Autodesk Fusion 360 part; units mm, degrees
(part 2 of 2)
sketch "Sketch38" plane through (0, 15.0006, 0) normal (0, -1, 0) x (1, 0, 0)
  line L0 (-1.1388, 9) -> (-3.0388, 9)
  line L1 (-3.0388, 9) -> (-3.0388, 0.2)
  line L2 (-3.0388, 0.2) -> (-3.0388, -5)
  line L3 (-3.0388, -5) -> (-1.1388, -5)
  line L4 (-1.1388, -5) -> (-1.1388, 9)
  line L5 (-3.7888, -3) -> (-3.0388, -3)
  line L6 (-3.0388, -3) -> (-3.0388, -5)
  line L7 (-3.0388, -5) -> (-3.7888, -3)
  line L8 (61.4612, 9) -> (59.5612, 9)
  line L9 (59.5612, 9) -> (59.5612, -5)
  line L10 (59.5612, -5) -> (61.4612, -5)
  line L11 (61.4612, -5) -> (61.4612, -1.4)
  line L12 (61.4612, -1.4) -> (61.4612, 9)
  line L13 (62.2112, -3) -> (61.4612, -3)
  line L14 (61.4612, -3) -> (61.4612, -5)
  line L15 (61.4612, -5) -> (62.2112, -3)
  dimension "d420" = 2
  dimension "d422" = 2
  constraint horizontal L5
  constraint vertical L6
  constraint coincident L2.end L3.start
  constraint horizontal L13
  constraint vertical L14
  constraint coincident L10.end L11.start
  measures "d420" distance of L2.end L5.end
  measures "d422" distance of L10.end L13.end
extrude "Extrude62" add sketch "Sketch38" against normal up to surface (8 mm away) contours L2 L5 L6 L7 | L11 L13 L14 L15 bodies 2
sketch "Sketch39" plane through (4.9612, 0, 0) normal (-1, 0, 0) x (0, -1, 0)
  line L0 (-52.9006, 9) -> (-54.8006, 9)
  line L1 (-54.8006, 9) -> (-54.8006, 0.2)
  line L2 (-54.8006, 0.2) -> (-54.8006, -5)
  line L3 (-54.8006, -5) -> (-52.9006, -5)
  line L4 (-52.9006, -5) -> (-52.9006, 9)
  line L5 (-55.5506, -3) -> (-54.8006, -3)
  line L6 (-54.8006, -3) -> (-54.8006, -5)
  line L7 (-54.8006, -5) -> (-55.5506, -3)
  dimension "d426" = 2
  constraint horizontal L5
  constraint vertical L6
  constraint coincident L2.end L3.start
  measures "d426" distance of L2.end L5.end
extrude "Extrude63" add sketch "Sketch39" against normal up to surface (8 mm away) contours L2 L5 L6 L7 bodies 2
sketch "Sketch40" plane through (53.4612, 0, 0) normal (1, 0, 0) x (0, 1, 0)
  line L0 (54.8006, 9) -> (52.9006, 9)
  line L1 (52.9006, 9) -> (52.9006, -5)
  line L2 (52.9006, -5) -> (54.8006, -5)
  line L3 (54.8006, -5) -> (54.8006, 0.2)
  line L4 (54.8006, 0.2) -> (54.8006, 9)
  line L5 (55.5506, -3) -> (54.8006, -3)
  line L6 (54.8006, -3) -> (54.8006, -5)
  line L7 (54.8006, -5) -> (55.5506, -3)
  dimension "d430" = 2
  constraint horizontal L5
  constraint vertical L6
  constraint coincident L2.end L3.start
  measures "d430" distance of L2.end L5.end
extrude "Extrude64" add sketch "Sketch40" against normal up to surface (8 mm away) contours L3 L5 L6 L7 bodies 2
sketch "Sketch41" plane through (0, 54.8006, 0) normal (0, -1, 0) x (1, 0, 0)
  line L0 (-2.0388, -7) -> (60.4612, -7)
  line L1 (60.4612, -7) -> (60.4612, -1.6)
  line L2 (60.4612, -1.6) -> (-2.0388, -1.6)
  line L3 (-2.0388, -1.6) -> (-2.0388, -7)
  line L4 (53.4612, -5) -> (53.4612, -3)
  line L5 (53.4612, -3) -> (45.4612, -3)
  line L6 (45.4612, -5) -> (45.4612, -3)
  line L7 (45.4612, -5) -> (53.4612, -5)
  line L8 (12.9612, -3) -> (12.9612, -5)
  line L9 (4.9612, -5) -> (12.9612, -5)
  line L10 (4.9612, -3) -> (12.9612, -3)
  line L11 (4.9612, -5) -> (4.9612, -3)
  line L12 (13.4612, -2.75) -> (4.4612, -2.75)
  line L13 (4.4612, -2.75) -> (4.4612, -5.5)
  line L14 (4.4612, -5.5) -> (13.4612, -5.5)
  line L15 (13.4612, -5.5) -> (13.4612, -2.75)
  line L16 (53.9612, -2.75) -> (44.9612, -2.75)
  line L17 (44.9612, -2.75) -> (44.9612, -5.5)
  line L18 (44.9612, -5.5) -> (53.9612, -5.5)
  line L19 (53.9612, -5.5) -> (53.9612, -2.75)
  dimension "d434" = 0.25
  dimension "d435" = 0.5
  dimension "d436" = 0.5
  dimension "d437" = 0.5
  dimension "d438" = 0.25
  dimension "d439" = 0.5
  dimension "d440" = 0.5
  dimension "d441" = 0.5
  constraint horizontal L12
  constraint vertical L13
  constraint horizontal L14
  constraint vertical L15
  constraint horizontal L16
  constraint vertical L17
  constraint horizontal L18
  constraint vertical L19
  measures "d434" distance of L10 L12
  measures "d435" distance of L9 L14
  measures "d436" distance of L8 L15
  measures "d437" distance of L11 L13
  measures "d438" distance of L5 L16
  measures "d439" distance of L6 L17
  measures "d440" distance of L7 L18
  measures "d441" distance of L4 L19
extrude "Extrude65" cut sketch "Sketch41" against normal blind 1 contours L4 L5 L6 L7 | L8 L9 L10 L11 | L12 L13 L14 L15 | L16 L17 L18 L19 bodies 1
sketch "Sketch42" plane through (61.4612, 0, 0) normal (-1, 0, 0) x (0, -1, 0)
  line L0 (-48.8006, -7) -> (-11.7006, -7)
  line L1 (-11.7006, -7) -> (-11.7006, -1.6)
  line L2 (-11.7006, -1.6) -> (-48.8006, -1.6)
  line L3 (-48.8006, -1.6) -> (-48.8006, -7)
  line L4 (-15.0006, -5) -> (-15.0006, -3)
  line L5 (-15.0006, -3) -> (-23.0006, -3)
  line L6 (-23.0006, -5) -> (-23.0006, -3)
  line L7 (-23.0006, -5) -> (-15.0006, -5)
  line L8 (-14.5006, -2.75) -> (-23.5006, -2.75)
  line L9 (-23.5006, -2.75) -> (-23.5006, -5.5)
  line L10 (-23.5006, -5.5) -> (-14.5006, -5.5)
  line L11 (-14.5006, -5.5) -> (-14.5006, -2.75)
  dimension "d444" = 0.25
  dimension "d445" = 0.5
  dimension "d446" = 0.5
  dimension "d447" = 0.5
  constraint horizontal L8
  constraint vertical L9
  constraint horizontal L10
  constraint vertical L11
  measures "d444" distance of L5 L8
  measures "d445" distance of L7 L10
  measures "d446" distance of L6 L9
  measures "d447" distance of L4 L11
extrude "Extrude66" cut sketch "Sketch42" against normal blind 1 contours L4 L5 L6 L7 | L8 L9 L10 L11 bodies 1
sketch "Sketch43" plane through (-3.0388, 0, 0) normal (1, 0, 0) x (0, 1, 0)
  line L0 (11.7006, -7) -> (48.8006, -7)
  line L1 (48.8006, -7) -> (48.8006, -1.6)
  line L2 (48.8006, -1.6) -> (11.7006, -1.6)
  line L3 (11.7006, -1.6) -> (11.7006, -7)
  line L4 (23.0006, -3) -> (23.0006, -5)
  line L5 (15.0006, -3) -> (23.0006, -3)
  line L6 (15.0006, -5) -> (15.0006, -3)
  line L7 (15.0006, -5) -> (23.0006, -5)
  line L8 (23.5006, -2.75) -> (14.5006, -2.75)
  line L9 (14.5006, -2.75) -> (14.5006, -5.5)
  line L10 (14.5006, -5.5) -> (23.5006, -5.5)
  line L11 (23.5006, -5.5) -> (23.5006, -2.75)
  dimension "d450" = 0.5
  dimension "d451" = 0.5
  dimension "d452" = 0.5
  dimension "d453" = 0.25
  constraint horizontal L8
  constraint vertical L9
  constraint horizontal L10
  constraint vertical L11
  measures "d450" distance of L6 L9
  measures "d451" distance of L7 L10
  measures "d452" distance of L4 L11
  measures "d453" distance of L5 L8
extrude "Extrude67" cut sketch "Sketch43" against normal blind 1 contours L4 L5 L6 L7 | L8 L9 L10 L11 bodies 1
copy_body "Body->Comp6" bodies 1 removing the originals makes body 3 in component "bottom shell"
copy_body "Body->Comp7" bodies 2 removing the originals makes body 4 in component "top shell"
sketch "Sketch44" plane through (63.4612, 0, 0) normal (1, 0, 0) x (0, 1, 0)
  line L0 (0.0006, -9) -> (53.8006, -9)
  line L1 (53.8006, -9) -> (53.8006, 0)
  line L2 (53.8006, 0) -> (0.0006, 0)
  line L3 (0.0006, 0) -> (0.0006, -9)
  line L4 (23.5006, -5.5) -> (23.5006, -2.75)
  line L5 (14.5006, -2.75) -> (14.5006, -5.5)
  line L6 (23.5006, -4.125) -> (14.5006, -4.125)
  point P0 (19.0006, -4.125)
  constraint midpoint L4 L6.start
  constraint midpoint L5 L6.end
  constraint midpoint L6 P0
hole "Hole1" at (63.4612, 19.0006, -4.125) direction (-1, 0, 0) diameter 2 depth 2 tip angle 180 bodies 3 in component "bottom shell"
sketch "Sketch45" plane through (-5.0388, 0, 0) normal (-1, 0, 0) x (0, -1, 0)
  line L0 (-53.8006, -9) -> (-0.0006, -9)
  line L1 (-0.0006, -9) -> (-0.0006, 0)
  line L2 (-0.0006, 0) -> (-53.8006, 0)
  line L3 (-53.8006, 0) -> (-53.8006, -9)
  line L4 (-14.5006, -5.5) -> (-14.5006, -2.75)
  line L5 (-23.5006, -2.75) -> (-23.5006, -5.5)
  line L6 (-23.5006, -4.125) -> (-14.5006, -4.125)
  point P0 (-19.0006, -4.125)
  constraint midpoint L5 L6.start
  constraint midpoint L4 L6.end
  constraint midpoint L6 P0
hole "Hole2" at (-5.0388, 19.0006, -4.125) direction (1, 0, 0) diameter 2 depth 2 tip angle 180 bodies 3 in component "bottom shell"
sketch "Sketch46" plane through (0, 56.8006, 0) normal (0, 1, 0) x (-1, 0, 0)
  line L0 (-60.4612, -9) -> (2.0388, -9)
  line L1 (2.0388, -9) -> (2.0388, 0)
  line L2 (2.0388, 0) -> (-60.4612, 0)
  line L3 (-60.4612, 0) -> (-60.4612, -9)
  line L4 (-13.4612, -2.75) -> (-13.4612, -5.5)
  line L5 (-4.4612, -5.5) -> (-4.4612, -2.75)
  line L6 (-53.9612, -2.75) -> (-53.9612, -5.5)
  line L7 (-44.9612, -5.5) -> (-44.9612, -2.75)
  line L8 (-53.9612, -4.125) -> (-44.9612, -4.125)
  line L9 (-13.4612, -4.125) -> (-4.4612, -4.125)
  point P0 (-8.9612, -4.125)
  point P1 (-49.4612, -4.125)
  constraint midpoint L6 L8.start
  constraint midpoint L7 L8.end
  constraint midpoint L4 L9.start
  constraint midpoint L5 L9.end
  constraint midpoint L9 P0
  constraint midpoint L8 P1
hole "Hole3" at (49.4612, 56.8006, -4.125) at (8.9612, 56.8006, -4.125) direction (0, -1, 0) diameter 2 depth 2 tip angle 180 bodies 3 in component "bottom shell"
fillet "Fillet1" radius 1 1 faces at (29.124, 23.0039, 9) on bodies 4 in component "top shell"
sketch "Sketch47" plane through (0, 9.7006, 0) normal (0, -1, 0) x (1, 0, 0)
  line L0 (-3.0388, -7) -> (61.4612, -7)
  line L1 (61.4612, -7) -> (61.4612, -1.6)
  line L2 (61.4612, -1.6) -> (61.4612, 0)
  line L3 (61.4612, 0) -> (58.6712, 0)
  line L4 (58.6712, 0) -> (58.6712, -1.6)
  line L5 (58.6712, -1.6) -> (-0.2488, -1.6)
  line L6 (-0.2488, -1.6) -> (-0.2488, 0)
  line L7 (-0.2488, 0) -> (-3.0388, 0)
  line L8 (-3.0388, 0) -> (-3.0388, -1.6)
  line L9 (-3.0388, -1.6) -> (-3.0388, -7)
  line L10 (61.4612, -1.6) -> (60.9612, -1.6)
  line L11 (60.9612, -1.6) -> (60.9612, 0)
  line L12 (60.9612, 0) -> (61.4612, -1.6)
  line L13 (-3.0388, -1.6) -> (-2.5388, -1.6)
  line L14 (-2.5388, -1.6) -> (-2.5388, 0)
  line L15 (-2.5388, 0) -> (-3.0388, -1.6)
  dimension "d466" = 0.5
  dimension "d467" = 0.5
  constraint horizontal L10
  constraint vertical L11
  constraint coincident L1.end L2.start
  constraint horizontal L13
  constraint vertical L14
  constraint coincident L8.end L9.start
  measures "d466" distance of L1.end L10.end
  measures "d467" distance of L8.end L13.end
extrude "Extrude1" cut sketch "Sketch47" against normal up to surface (2 mm away) contours L7 L8 L15 | L2 L3 L12 bodies 3 in component "bottom shell"
component "bottom shell" placed x (1, 0, 0) y (0, 1, 0) z (0, 0, 1) at (0, 0, 0)
component "top shell" placed x (1, 0, 0) y (0, 1, 0) z (0, 0, 1) at (0, 0, 0)
equation "d76 = Top_Plane_Offset"
equation "d80 = Top_Case_Height"
equation "d96 = d88"
equation "d97 = d87"
equation "d282 = d87"
equation "d283 = d88"
equation "d284 = d87"
equation "d285 = d88"
equation "d287 = d286"
equation "Top_Plane_Offset = 11 mm"
equation "Top_Case_Height = -( Top_Plane_Offset - 0.2 mm )"
equation "Top_Case_Lip_Height = 1.6 mm"
equation "d387 = d386"
equation "d392 = Top_Case_Lip_Height"
equation "d396 = Top_Case_Post_Height"
equation "Top_Case_Post_Height = 8.5 mm"
equation "d400 = Top_Cast_Post_Lip"
equation "d411 = d410"
equation "d413 = d412"
equation "Top_Case_Tab_Length = 14 mm"
equation "d415 = Top_Case_Tab_Length"
equation "Top_Cast_Post_Lip = 1.5 mm"
named bodies: "bottom shell", "top shell"
